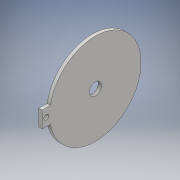
# Autodesk Inventor part: toppart
Saved by Autodesk Inventor 2018 (Build 220112000, 112)
## iProperties
Created: 2019-10-09
Part Number: toppart
Material: 一般
Document SubType Name: Modeling
Designer: Eiji Nishizawa
Density: 1 g/cm^3
Appearance: 既定
Author: Eiji Nishizawa
Autodesk Inventor part; units mm, degrees
ref_plane "YZ Plane" through (0, 0, 0) normal (1, 0, 0) x (0, 1, 0)
ref_plane "XZ Plane" through (0, 0, 0) normal (0, 1, 0) x (-1, 0, 0)
ref_plane "XY Plane" through (0, 0, 0) normal (0, 0, 1) x (1, 0, 0)
sketch "スケッチ1" plane through (0, 0, 0) normal (1, 0, 0) x (0, 1, 0)
  circle A0 centre (0, 0) radius 28
  circle A1 centre (0, 0) radius 3.75
  line L0 (-32.55, 5) -> (-27.55, 5)
  line L1 (-27.55, 5) -> (-27.55, -5)
  line L2 (-27.55, -5) -> (-32.55, -5)
  line L3 (-32.55, -5) -> (-32.55, 5)
  line L4 (-32.55, 5) -> (-27.55, -5) construction
  line L5 (-27.55, 5) -> (-32.55, -5) construction
  circle A2 centre (-30.05, 0) radius 1.5
  dimension "d1" = 56
  dimension "d0" = 7.5
  dimension "d2" = 10
  dimension "d3" = 5
  dimension "d4" = 0
  dimension "d5" = 3
  constraints: 12 end point, 3 coincident, 2 centre point, 2 midpoint, 2 parallel, 1 horizontal, 1 perpendicular, 3 other
  measures "d0" diameter of A1
  measures "d2" distance of L2.end L0.start
  measures "d3" distance of L1.end L2.end
  measures "d4" vertical distance of point (0, 0) point (-30.05, 0)
  measures "d5" diameter of A2
extrude "押し出し1" add sketch "スケッチ1" along normal blind 2
